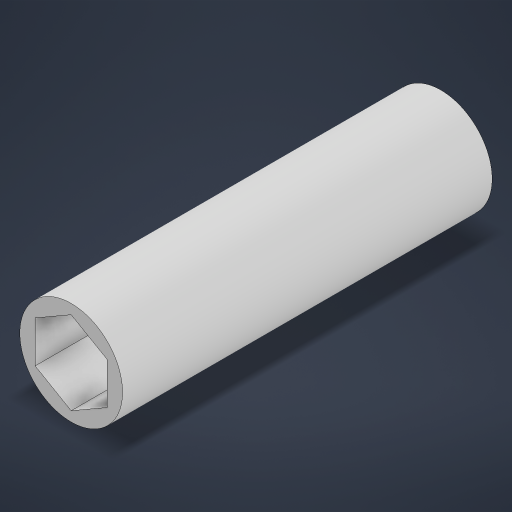
# Autodesk Inventor part: TestingWinch
Saved by Autodesk Inventor 2024 (Build 280153000, 153)
## iProperties
Created: 2024-03-11
Part Number: TestingWinch
Material: Generic
Document SubType Name: Modeling
Designer: avsar
Density: 1 g/cm^3
Appearance: Default
Author: avsar
Autodesk Inventor part; units mm, degrees
ref_plane "YZ Plane" through (0, 0, 0) normal (1, 0, 0) x (0, 1, 0)
ref_plane "XZ Plane" through (0, 0, 0) normal (0, 1, 0) x (-1, 0, 0)
ref_plane "XY Plane" through (0, 0, 0) normal (0, 0, 1) x (1, 0, 0)
sketch "Sketch1" plane through (0, 0, 0) normal (0, 0, 1) x (1, 0, 0)
  arc A0 (-4.5, -2.1795) -> (-4.5, 2.1795) centre (0, 0) ccw
  line L0 (-4.5, 2.1795) -> (-4.5, -2.1795)
  arc A1 (-4.5, 2.1795) -> (-4.5, -2.1795) centre (0, 0) ccw construction
  arc A2 (-4.6, -2.2023) -> (-4.6, 2.2023) centre (0, 0) ccw construction
  line L1 (-4.6, -2.2023) -> (-4.6, 2.2023) construction
  circle A3 centre (0, 0) radius 8 construction
  dimension "d0" = 10
  dimension "d1" = 4.359
  dimension "d2" = 0.1
  dimension "d3" = 16
  constraints: 6 point on circle, 4 centre point, 4 end point, 3 coincident, 1 vertical, 1 other
  measures "d0" diameter of A0
  measures "d1" distance of L0.start L0.end
  measures "d2" radial gap between concentric circles of A0 A2
  measures "d3" diameter of A3
extrude "Extrusion1" add sketch "Sketch1" along normal blind 24
sketch "Sketch3" plane through (0, 0, 24) normal (0, 0, 1) x (1, 0, 0)
  circle A0 centre (0, 0) radius 5
  circle A1 centre (0, 0) radius 4.05 construction
  line L0 (0, 0) -> (0, 4.05) construction
  line L1 (0, 4.05) -> (3.5074, 2.025)
  line L2 (3.5074, 2.025) -> (3.5074, -2.025)
  line L3 (0, -4.05) -> (3.5074, -2.025)
  line L4 (0, -4.05) -> (-3.5074, -2.025)
  line L5 (-3.5074, -2.025) -> (-3.5074, 2.025)
  line L6 (-3.5074, 2.025) -> (0, 4.05)
  point P0 (-4.5, 2.1795)
  dimension "d15" = 8.1
  constraints: 14 end point, 6 point on circle, 3 parallel, 2 coincident, 1 centre point, 1 equal length, 1 point on line, 1 vertical, 3 other
  measures "d15" diameter of A1
extrude "Extrusion4" add sketch "Sketch3" along normal blind 12
body "Solid1"
